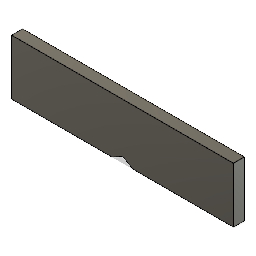
Table_17p1_Problem_4 (Autodesk Fusion 360 design; units mm, degrees)
Autodesk Fusion 360 part; units mm, degrees
sketch "Sketch1" plane through (0, 0, 0) normal (0, 0, 1) x (1, 0, 0)
  line L0 (-100, 0) -> (-100, 25)
  line L1 (-100, 25) -> (100, 25)
  line L2 (100, 25) -> (100, 0)
  line L3 (100, 0) -> (100, -25)
  line L4 (100, -25) -> (9.3301, -25)
  line L5 (9.3301, -25) -> (1.25, -20.3349)
  arc A0 (1.25, -20.3349) -> (-1.25, -20.3349) centre (0, -22.5) ccw
  line L6 (-1.25, -20.3349) -> (-9.3301, -25)
  line L7 (-9.3301, -25) -> (-100, -25)
  line L8 (-100, -25) -> (-100, 0)
  line L9 (-100, 0) -> (100, 0) construction
  line L10 (0, 0) -> (0, -22.5) construction
  line L11 (-100, -20) -> (100, -20) construction
  dimension "Total_Width" = 200
  dimension "Total_Height" = 50
  dimension "Notch_Radius" = 2.5
  dimension "Notch_Theta" = 120
  dimension "Notch_Height" = 5
  constraint vertical L0
  constraint perpendicular L0 L1
  constraint perpendicular L1 L2
  constraint perpendicular L1 L3
  constraint perpendicular L3 L4
  constraint tangent L5 A0
  constraint tangent A0 L6
  constraint parallel L4 L7
  constraint perpendicular L7 L8
  constraint equal L0 L8
  constraint equal L3 L8
  constraint equal L0 L2
  constraint coincident L10.start origin
  constraint coincident A0.centre L10.end
  constraint perpendicular L9 L10
  constraint coincident L8 L11.start
  constraint coincident L3 L11.end
  constraint horizontal L11
  constraint tangent A0 L11
  constraint equal L5 L6
  constraint coincident L10.start L9
  constraint equal L4 L7
  measures "Total_Width" distance of L0.end L1.end
  measures "Total_Height" distance of L1 L7
  measures "Notch_Radius" radius of A0
  measures "Notch_Theta" angle of L5 L6
  measures "Notch_Height" distance of L7 L11
extrude "Extrude1" add sketch "Sketch1" along normal mid plane 10
equation "Thickness = 1 cm"
